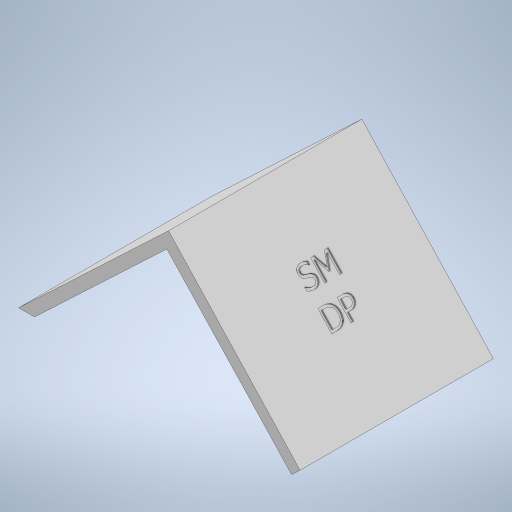
# Autodesk Inventor part: Escritura
Saved by Autodesk Inventor 2023 (Build 270158000, 158)
## iProperties
Created: 2022-08-26
Part Number: Escritura
Material: Generic
Document SubType Name: Modeling
Designer: SAMJ
Density: 1 g/cm^3
Appearance: Default
Author: SAMJ
Autodesk Inventor part; units mm, degrees
ref_plane "YZ Plane" through (0, 0, 0) normal (1, 0, 0) x (0, 1, 0)
ref_plane "XZ Plane" through (0, 0, 0) normal (0, 1, 0) x (-1, 0, 0)
ref_plane "XY Plane" through (0, 0, 0) normal (0, 0, 1) x (1, 0, 0)
sketch "Sketch1" plane through (0, 0, 0) normal (0, 0, 1) x (1, 0, 0)
  line L0 (0, 0) -> (39.2, 0)
  line L1 (0, 0) -> (412, 0) construction
  line L2 (0, 0) -> (219.498, 207.4238)
  line L3 (0, 0) -> (302, 0) construction
  line L4 (219.498, 207.4238) -> (412, 0)
  line L5 (0, 0) -> (10.9893, -11.629)
  line L6 (412, 0) -> (399.5998, -11.629)
  line L7 (10.9893, -11.629) -> (217.0153, 183.0638)
  line L8 (217.0153, 183.0638) -> (399.5998, -11.629)
  point P0 (23.2953, 0)
  dimension "d1" = 412
  dimension "d2" = 302
  dimension "d3" = 43.38
  dimension "d4" = 16
  dimension "d5" = 17
  constraints: 18 end point, 3 horizontal, 2 perpendicular, 1 equal length
  measures "d1" distance of L0.start L1.end
  measures "d2" distance of L0.start L2.end
  measures "d3" angle of L3 L2
  measures "d4" distance of L0.start L5.end
  measures "d5" distance of L1.end L6.end
extrude "Extrusion1" add sketch "Sketch1" against normal blind 283 contours L2 L4 L6 L8 L7 L0
sketch "Sketch2" plane through (412, 0, 0) normal (0.7329799, 0.6802503, 0) x (0, 0, -1)
  line L0 (115.4319, 185.8061) -> (173.3744, 185.8061) construction
  line L1 (173.3744, 185.8061) -> (173.3744, 105.877) construction
  line L2 (173.3744, 105.877) -> (115.4319, 105.877) construction
  line L3 (115.4319, 105.877) -> (115.4319, 185.8061) construction
  spline S0 degree 2 poles (126.8338, 154.7364) (123.5761, 154.7364) (119.0056, 156.0978) (116.9878, 157.0703) knots 0 0 0 1 2 2 2
  line L4 (116.9878, 157.0703) -> (116.9878, 162.0784)
  line L5 (116.9878, 162.0784) -> (117.2795, 162.0784)
  spline S1 degree 2 poles (117.2795, 162.0784) (119.2487, 160.2307) (124.2325, 158.1886) (126.5421, 158.1886) knots 0 0 0 1 2 2 2
  spline S2 degree 2 poles (126.5421, 158.1886) (129.8484, 158.1886) (133.2277, 160.9358) (133.2277, 163.1967) knots 0 0 0 1 2 2 2
  spline S3 degree 2 poles (133.2277, 163.1967) (133.2277, 164.9957) (131.453, 167.2324) (129.5324, 167.7915) knots 0 0 0 1 2 2 2
  spline S4 degree 2 poles (129.5324, 167.7915) (128.1466, 168.1805) (125.8371, 168.7153) (124.111, 169.1529) knots 0 0 0 1 2 2 2
  spline S5 degree 2 poles (124.111, 169.1529) (122.5551, 169.5662) (120.0996, 170.8061) (119.1515, 171.8029) knots 0 0 0 1 2 2 2
  spline S6 degree 2 poles (119.1515, 171.8029) (118.2277, 172.7996) (117.2066, 175.4739) (117.2066, 177.2243) knots 0 0 0 1 2 2 2
  spline S7 degree 2 poles (117.2066, 177.2243) (117.2066, 180.8709) (122.8954, 185.8061) (127.2957, 185.8061) knots 0 0 0 1 2 2 2
  spline S8 degree 2 poles (127.2957, 185.8061) (129.8241, 185.8061) (134.2974, 184.8093) (136.2179, 183.8612) knots 0 0 0 1 2 2 2
  line L6 (136.2179, 183.8612) -> (136.2179, 179.0962)
  line L7 (136.2179, 179.0962) -> (135.9262, 179.0962)
  spline S9 degree 2 poles (135.9262, 179.0962) (134.4919, 180.409) (130.0186, 182.3539) (127.5632, 182.3539) knots 0 0 0 1 2 2 2
  spline S10 degree 2 poles (127.5632, 182.3539) (124.7917, 182.3539) (121.3638, 179.7526) (121.3638, 177.6375) knots 0 0 0 1 2 2 2
  spline S11 degree 2 poles (121.3638, 177.6375) (121.3638, 175.7413) (123.3816, 173.4803) (125.2779, 172.9698) knots 0 0 0 1 2 2 2
  spline S12 degree 2 poles (125.2779, 172.9698) (126.5421, 172.6294) (130.2131, 171.7542) (131.4286, 171.3896) knots 0 0 0 1 2 2 2
  spline S13 degree 2 poles (131.4286, 171.3896) (134.5162, 170.4414) (137.3849, 166.6246) (137.3849, 163.8288) knots 0 0 0 1 2 2 2
  spline S14 degree 2 poles (137.3849, 163.8288) (137.3849, 162.0541) (135.9505, 158.6505) (134.662, 157.4593) knots 0 0 0 1 2 2 2
  spline S15 degree 2 poles (134.662, 157.4593) (133.2277, 156.1465) (129.581, 154.7364) (126.8338, 154.7364) knots 0 0 0 1 2 2 2
  line L8 (167.1661, 155.2713) -> (163.1791, 155.2713)
  line L9 (163.1791, 155.2713) -> (163.1791, 181.114)
  line L10 (163.1791, 181.114) -> (155.3509, 163.5371)
  line L11 (155.3509, 163.5371) -> (152.9197, 163.5371)
  line L12 (152.9197, 163.5371) -> (145.1645, 181.114)
  line L13 (145.1645, 181.114) -> (145.1645, 155.2713)
  line L14 (145.1645, 155.2713) -> (141.4449, 155.2713)
  line L15 (141.4449, 155.2713) -> (141.4449, 185.2713)
  line L16 (141.4449, 185.2713) -> (146.8906, 185.2713)
  line L17 (146.8906, 185.2713) -> (154.3784, 168.5695)
  line L18 (154.3784, 168.5695) -> (161.6231, 185.2713)
  line L19 (161.6231, 185.2713) -> (167.1661, 185.2713)
  line L20 (167.1661, 185.2713) -> (167.1661, 155.2713)
  spline S16 degree 2 poles (142.1256, 120.8527) (142.1256, 116.7441) (138.7949, 110.1315) (135.9991, 108.2839) knots 0 0 0 1 2 2 2
  spline S17 degree 2 poles (135.9991, 108.2839) (133.7139, 106.8495) (129.0218, 105.877) (125.3752, 105.877) knots 0 0 0 1 2 2 2
  line L21 (125.3752, 105.877) -> (118.4708, 105.877)
  line L22 (118.4708, 105.877) -> (118.4708, 135.877)
  line L23 (118.4708, 135.877) -> (125.3022, 135.877)
  spline S18 degree 2 poles (125.3022, 135.877) (129.5324, 135.877) (134.346, 134.6129) (136.0478, 133.4945) knots 0 0 0 1 2 2 2
  spline S19 degree 2 poles (136.0478, 133.4945) (138.9408, 131.574) (142.1256, 125.2287) (142.1256, 120.8527) knots 0 0 0 1 2 2 2
  spline S20 degree 2 poles (137.9684, 120.9014) (137.9684, 124.3535) (135.6831, 129.2401) (133.4222, 130.6258) knots 0 0 0 1 2 2 2
  spline S21 degree 2 poles (133.4222, 130.6258) (131.8176, 131.574) (128.1953, 132.4249) (125.4967, 132.4249) knots 0 0 0 1 2 2 2
  line L24 (125.4967, 132.4249) -> (122.4578, 132.4249)
  line L25 (122.4578, 132.4249) -> (122.4578, 109.3292)
  line L26 (122.4578, 109.3292) -> (125.4967, 109.3292)
  spline S22 degree 2 poles (125.4967, 109.3292) (128.1466, 109.3292) (132.158, 110.1801) (133.7868, 111.3228) knots 0 0 0 1 2 2 2
  spline S23 degree 2 poles (133.7868, 111.3228) (135.8776, 112.7328) (137.9684, 117.4005) (137.9684, 120.9014) knots 0 0 0 1 2 2 2
  spline S24 degree 2 poles (165.4157, 126.8333) (165.4157, 124.8884) (164.0299, 121.3876) (162.7901, 120.172) knots 0 0 0 1 2 2 2
  spline S25 degree 2 poles (162.7901, 120.172) (161.2342, 118.6404) (157.0283, 117.0602) (153.8192, 117.0602) knots 0 0 0 1 2 2 2
  line L27 (153.8192, 117.0602) -> (150.44, 117.0602)
  line L28 (150.44, 117.0602) -> (150.44, 105.877)
  line L29 (150.44, 105.877) -> (146.453, 105.877)
  line L30 (146.453, 105.877) -> (146.453, 135.877)
  line L31 (146.453, 135.877) -> (153.9894, 135.877)
  spline S26 degree 2 poles (153.9894, 135.877) (156.6637, 135.877) (160.4076, 135.0018) (161.8419, 134.0051) knots 0 0 0 1 2 2 2
  spline S27 degree 2 poles (161.8419, 134.0051) (163.5194, 132.8625) (165.4157, 129.3373) (165.4157, 126.8333) knots 0 0 0 1 2 2 2
  spline S28 degree 2 poles (161.2585, 126.7117) (161.2585, 128.2676) (160.1888, 130.5529) (159.0948, 131.2822) knots 0 0 0 1 2 2 2
  spline S29 degree 2 poles (159.0948, 131.2822) (158.1466, 131.9143) (155.6183, 132.4249) (153.7463, 132.4249) knots 0 0 0 1 2 2 2
  line L32 (153.7463, 132.4249) -> (150.44, 132.4249)
  line L33 (150.44, 132.4249) -> (150.44, 120.4638)
  line L34 (150.44, 120.4638) -> (153.1628, 120.4638)
  spline S30 degree 2 poles (153.1628, 120.4638) (155.594, 120.4638) (158.5842, 121.2417) (159.5567, 122.2628) knots 0 0 0 1 2 2 2
  spline S31 degree 2 poles (159.5567, 122.2628) (160.4562, 123.1623) (161.2585, 125.2774) (161.2585, 126.7117) knots 0 0 0 1 2 2 2
  point P0 (0, 280.2631)
  constraints: 2 other
extrude "Extrusion2" cut sketch "Sketch2" against normal blind 2
body "Solid1"
